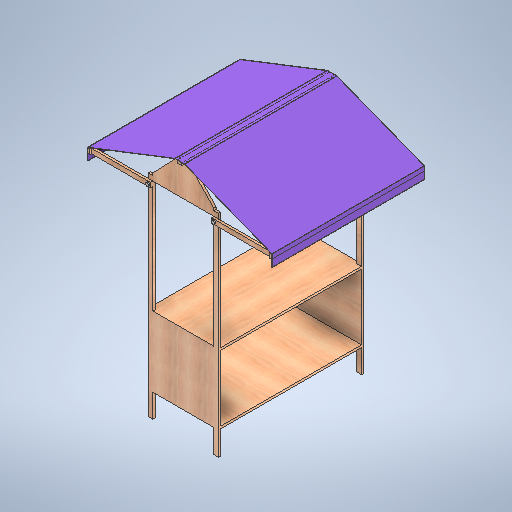
# Autodesk Inventor part: Pieza1
Saved by Autodesk Inventor 2025 (Build 290162000, 162)
## iProperties
Created: 2024-07-07
Part Number: Pieza1
Material: Genérico
Document SubType Name: Modeling
Designer: USER
Density: 1 g/cm^3
Appearance: Valor por defecto
Finish7_Appearance: Birch - Natural Medium Gloss
Finish7_Area: 449600,000 mm^2
Finish1_Appearance: Birch - Natural Polished
Finish1_Area: 7576908,613 mm^2
Finish2_Appearance: Aluminum - Polished
Finish2_Area: 5463,586 mm^2
Finish3_Appearance: Birch - Natural Polished
Finish3_Area: 400,000 mm^2
Finish4_Appearance: Birch - Natural Polished
Finish4_Area: 4880,000 mm^2
Finish5_Appearance: Birch - Natural Polished
Finish5_Area: 6080,000 mm^2
Finish6_Appearance: Violet
Finish6_Process: Prime/Paint RAL 3018
Finish6_Description: Prima/pintura RAL 3018
Finish6_ShortDescription: RAL 3018
Finish6_Thickness: 0,050 mm
Finish6_Area: 4778797,792 mm^2
Author: USER
Autodesk Inventor part; units mm, degrees
ref_plane "YZ Plane" through (0, 0, 0) normal (1, 0, 0) x (0, 1, 0)
ref_plane "XZ Plane" through (0, 0, 0) normal (0, 1, 0) x (-1, 0, 0)
ref_plane "XY Plane" through (0, 0, 0) normal (0, 0, 1) x (1, 0, 0)
sketch "Boceto1" plane through (0, 0, 0) normal (0, 1, 0) x (-1, 0, 0)
  line L0 (0, 0) -> (600, 0)
  line L1 (600, 0) -> (600, -1240)
  line L2 (600, -1240) -> (0, -1240)
  line L3 (0, -1240) -> (0, 0)
  dimension "d0" = 600
  dimension "d1" = 1240
  constraints: 8 end point, 2 parallel, 1 horizontal, 1 perpendicular
  measures "d0" distance of L1.end L2.end
  measures "d1" distance of L0.end L1.end
extrude "Extrusión1" add sketch "Boceto1" along normal blind 1800
sketch "Boceto2" plane through (-600, 0, 0) normal (0, 0, 1) x (1, 0, 0)
  line L0 (600, 0) -> (0, 0) projected
  line L1 (0, 0) -> (40, 0)
  line L2 (40, 0) -> (40, 200)
  line L3 (600, 0) -> (560, 0)
  line L4 (560, 0) -> (560, 200)
  line L5 (40, 200) -> (560, 200)
  line L6 (560, 200) -> (560, 0)
  line L7 (560, 0) -> (40, 0)
  line L8 (40, 0) -> (40, 200)
  line L9 (40, 200) -> (560, 200)
  line L10 (560, 800) -> (40, 800)
  line L11 (600, 1800) -> (0, 1800) projected
  line L12 (40, 800) -> (560, 800)
  line L13 (560, 800) -> (560, 1800)
  line L14 (560, 1800) -> (40, 1800)
  line L15 (40, 1800) -> (40, 800)
  dimension "d5" = 200
  dimension "d7" = 200
  dimension "d9" = 520
  constraints: 28 end point, 5 horizontal, 5 parallel, 4 perpendicular, 2 point on line
  measures "d5" distance of L2.end L1.end
  measures "d7" distance of L3.end L4.end
  measures "d9" distance of L14.end L13.end
extrude "Extrusión2" cut sketch "Boceto2" against normal blind 1240
sketch "Boceto3" plane through (0, 0, 0) normal (1, 0, 0) x (0, 0, -1)
  line L0 (0, 0) -> (20, 0)
  line L1 (20, 0) -> (20, 200)
  line L2 (20, 200) -> (0, 200)
  line L3 (0, 200) -> (0, 0)
  line L4 (0, 0) -> (1240, 0) projected
  line L5 (1240, 0) -> (1220, 0)
  line L6 (1220, 0) -> (1220, 200)
  line L7 (1220, 200) -> (1240, 200)
  line L8 (1240, 200) -> (1240, 0)
  line L9 (20, 200) -> (1220, 200)
  line L10 (1220, 200) -> (1220, 0)
  line L11 (1220, 0) -> (20, 0)
  line L12 (20, 0) -> (20, 200)
  line L13 (0, 800) -> (1240, 800) projected
  line L14 (20, 200) -> (1220, 200)
  line L15 (1220, 200) -> (1220, 780)
  line L16 (1220, 800) -> (20, 800)
  line L17 (20, 800) -> (20, 780)
  line L18 (20, 800) -> (1220, 800)
  line L19 (1220, 800) -> (1220, 780)
  line L20 (1220, 780) -> (20, 780)
  line L21 (20, 780) -> (20, 800)
  line L22 (20, 200) -> (1220, 200)
  line L23 (1220, 200) -> (1220, 220)
  line L24 (1220, 220) -> (20, 220)
  line L25 (20, 220) -> (20, 200)
  line L26 (0, 1800) -> (1240, 1800) projected
  line L27 (20, 800) -> (1220, 800)
  line L28 (1220, 800) -> (1220, 1800)
  line L29 (1220, 1800) -> (20, 1800)
  line L30 (20, 1800) -> (20, 800)
  line L31 (20, 780) -> (20, 220)
  line L32 (20, 220) -> (20, 200)
  line L33 (1220, 780) -> (1220, 800)
  dimension "d12" = 20
  dimension "d13" = 200
  dimension "d14" = 20
  dimension "d15" = 200
  dimension "d16" = 1200
  dimension "d17" = 20
  dimension "d18" = 1200
  dimension "d19" = 20
  dimension "d20" = 1200
  constraints: 62 end point, 19 parallel, 8 perpendicular, 7 horizontal, 2 point on line
  measures "d12" distance of L2.end L1.end
  measures "d13" distance of L1.end L0.end
  measures "d14" distance of L6.end L7.end
  measures "d15" distance of L5.end L6.end
  measures "d16" distance of L16.end L16.start
  measures "d17" distance of L18.end L15.end
  measures "d18" distance of L24.end L23.end
  measures "d19" distance of L23.end L22.end
  measures "d20" distance of L29.end L28.end
extrude "Extrusión3" cut sketch "Boceto3" against normal blind 600 contours L1 L9 L6 L4 | L30 L26 L28 L13
sketch "Boceto4" plane through (0, 0, -1240) normal (1, 0, 0) x (0, 0, -1)
  line L0 (-20, 800) -> (-20, 780)
  line L1 (-20, 780) -> (-1220, 780)
  line L2 (-1220, 780) -> (-1220, 800)
  line L3 (-20, 200) -> (-20, 220)
  line L4 (-20, 220) -> (-1220, 220)
  line L5 (-1220, 220) -> (-1220, 200)
  line L6 (-1220, 780) -> (-20, 780)
  line L7 (-20, 780) -> (-20, 220)
  line L8 (-20, 220) -> (-1220, 220)
  line L9 (-1220, 220) -> (-1220, 780)
  point P0 (-1240, 0)
  dimension "d23" = 1200
  dimension "d24" = 20
  dimension "d25" = 1200
  dimension "d26" = 20
  constraints: 20 end point, 4 parallel, 1 horizontal, 1 perpendicular
  measures "d23" distance of L0.end L1.end
  measures "d24" distance of L0.start L0.end
  measures "d25" distance of L4.end L3.end
  measures "d26" distance of L3.end L3.start
extrude "Extrusión4" cut sketch "Boceto4" against normal blind 580
sketch "Boceto5" plane through (0, 0, 0) normal (0, 0, 1) x (1, 0, 0)
  line L0 (0, 0) -> (0, 2050)
  line L1 (0, 0) -> (2050, 0) construction
  line L2 (0, 2050) -> (-560, 2050)
  line L3 (-560, 2050) -> (-560, 1760)
  line L4 (-560, 1760) -> (0, 1760)
  line L5 (0, 1760) -> (0, 2050)
  line L6 (0, 1760) -> (-40, 1760)
  line L7 (-40, 1760) -> (-40, 2050)
  line L8 (-40, 2050) -> (0, 2050)
  line L9 (0, 2050) -> (0, 1760)
  line L10 (-560, 1760) -> (-40, 1760)
  line L11 (-40, 1760) -> (-40, 1820)
  line L12 (-40, 1820) -> (-560, 1820)
  line L13 (-560, 1820) -> (-560, 1760)
  line L14 (-560, 2050) -> (-340, 2050)
  line L15 (-340, 2050) -> (-260, 2050)
  line L16 (-260, 2050) -> (-40, 1820)
  line L17 (-340, 2050) -> (-560, 1820)
  dimension "d29" = 2050
  dimension "d30" = 90
  dimension "d31" = 560
  dimension "d32" = 290
  dimension "d33" = 520
  dimension "d34" = 60
  dimension "d35" = 220
  dimension "d36" = 80
  constraints: 36 end point, 6 parallel, 4 horizontal, 4 perpendicular, 3 point on line, 1 vertical
  measures "d29" distance of L0.start L0.end
  measures "d30" angle of L1 L0
  measures "d31" distance of L4.end L3.end
  measures "d32" distance of L3.end L2.end
  measures "d33" distance of L12.end L11.end
  measures "d34" distance of L11.end L10.end
  measures "d35" distance of L2.end L14.end
  measures "d36" distance of L14.end L15.end
extrude "Extrusión5" add sketch "Boceto5" against normal blind 1240 contours L4 L3 L12 L7 | L12 L17 L2 L16
sketch "Boceto6" plane through (-40, 1760, -20) normal (1, 0, 0) x (0, 0, -1)
  line L0 (0, 0) -> (1200, 0) projected
  line L1 (-20, 290) -> (1220, 290) projected
  line L2 (0, 0) -> (1200, 0)
  line L3 (1200, 0) -> (1200, 290)
  line L4 (1200, 290) -> (0, 290)
  line L5 (0, 290) -> (0, 0)
  point P0 (-20, -1760)
  dimension "d39" = 1200
  constraints: 8 end point, 2 parallel, 1 horizontal, 1 perpendicular, 1 point on line
  measures "d39" distance of L4.end L3.end
extrude "Extrusión6" cut sketch "Boceto6" against normal blind 520
sketch "Boceto7" plane through (-600, 0, 0) normal (0, 0, 1) x (1, 0, 0)
  line L0 (40, 800) -> (40, 1760) projected
  line L1 (40, 1760) -> (-465, 1760)
  line L2 (-465, 1760) -> (-465, 1720)
  line L3 (-465, 1720) -> (40, 1720)
  line L4 (40, 1720) -> (40, 1760)
  line L5 (560, 1760) -> (560, 800) projected
  line L6 (560, 1760) -> (1065, 1760)
  line L7 (1065, 1760) -> (1065, 1720)
  line L8 (1065, 1720) -> (560, 1720)
  line L9 (560, 1720) -> (560, 1760)
  point P0 (600, 0)
  dimension "d42" = 505
  dimension "d43" = 40
  dimension "d44" = 505
  dimension "d45" = 40
  constraints: 16 end point, 4 parallel, 2 horizontal, 2 perpendicular
  measures "d42" distance of L3.end L2.end
  measures "d43" distance of L2.end L1.end
  measures "d44" distance of L7.end L8.end
  measures "d45" distance of L6.end L7.end
extrude "Extrusión7" add sketch "Boceto7" along normal blind 20 and the other way blind 1260
sketch "Boceto8" plane through (465, 1720, 20) normal (1, 0, 0) x (0, 0, -1)
  line L0 (20, 40) -> (0, 40) projected
  line L1 (1280, 0) -> (1260, 0) projected
  line L2 (20, 40) -> (1260, 40)
  line L3 (1260, 40) -> (1260, 0)
  line L4 (1260, 0) -> (20, 0)
  line L5 (20, 0) -> (20, 40)
  point P0 (20, -1720)
  constraints: 8 end point, 2 parallel, 1 horizontal, 1 perpendicular
extrude "Extrusión8" cut sketch "Boceto8" against normal blind 465
sketch "Boceto9" plane through (-1065, 1720, 20) normal (-1, 0, 0) x (0, 0, 1)
  line L0 (-20, 0) -> (-20, -920) projected
  line L1 (-1260, 40) -> (-1260, 80) projected
  line L2 (-20, 0) -> (-1260, 0)
  line L3 (-1260, 0) -> (-1260, 40)
  line L4 (-1260, 40) -> (-20, 40)
  line L5 (-20, 40) -> (-20, 0)
  point P0 (-20, -1720)
  constraints: 8 end point, 2 parallel, 1 horizontal, 1 perpendicular
extrude "Extrusión9" cut sketch "Boceto9" against normal blind 465
sketch "Boceto10" plane through (-600, 0, -1220) normal (-1, 0, 0) x (0, 0, 1)
  line L0 (0, 1760) -> (0, 1800) projected
  line L1 (0, 1720) -> (1200, 1720) projected
  line L2 (0, 1760) -> (1200, 1760)
  line L3 (1200, 1760) -> (1200, 1720)
  line L4 (1200, 1720) -> (0, 1720)
  line L5 (0, 1720) -> (0, 1760)
  point P0 (1220, 0)
  constraints: 8 end point, 2 parallel, 1 horizontal, 1 perpendicular
extrude "Extrusión10" cut sketch "Boceto10" against normal blind 600
sketch "Boceto11" plane through (-600, 0, -1260) normal (0, 0, -1) x (-1, 0, 0)
  line L0 (-560, 1760) -> (-560, 800) projected
  line L1 (-579.0242, 1739.1271) -> (-579.8656, 1739.9613)
  line L2 (-569.9328, 1749.9806) -> (-566.2222, 1736.3689)
  line L3 (-566.2222, 1736.3689) -> (-576.155, 1726.3495)
  line L4 (-576.155, 1726.3495) -> (-589.7984, 1729.9419)
  line L5 (-589.7984, 1729.9419) -> (-593.509, 1743.5536)
  line L6 (-593.509, 1743.5536) -> (-583.5762, 1753.573)
  line L7 (-583.5762, 1753.573) -> (-569.9328, 1749.9806)
  line L8 (-40, 1760) -> (-560, 1760) projected
  line L9 (0, 1760) -> (0, 1720) projected
  line L10 (-10, 1750) -> (-6.3397, 1736.3397)
  line L11 (-6.3397, 1736.3397) -> (-16.3397, 1726.3397)
  line L12 (-16.3397, 1726.3397) -> (-30, 1730)
  line L13 (-30, 1730) -> (-33.6603, 1743.6603)
  line L14 (-33.6603, 1743.6603) -> (-23.6603, 1753.6603)
  line L15 (-23.6603, 1753.6603) -> (-10, 1750)
  point P0 (-600, 0)
  point P1 (-20, 1740)
  constraints: 26 end point, 1 coincident, 26 other
extrude "Extrusión11" add sketch "Boceto11" along normal blind 10 and the other way blind 1290
sketch "Boceto12" plane through (-600, 800, -1220) normal (-1, 0, 0) x (0, 0, 1)
  line L0 (0, 1000) -> (0, 0) projected
  line L1 (1200, 960) -> (1200, 0) projected
  line L2 (0, 1000) -> (1200, 1000)
  line L3 (1200, 1000) -> (1200, 911.7503)
  line L4 (1200, 911.7503) -> (0, 911.7503)
  line L5 (0, 911.7503) -> (0, 1000)
  point P0 (1220, -800)
  constraints: 8 end point, 2 parallel, 1 horizontal, 1 perpendicular, 1 point on line
extrude "Extrusión12" cut sketch "Boceto12" against normal blind 600
sketch "Boceto13" plane through (-340, 2050, 0) normal (0, 0, 1) x (1, 0, 0)
  line L0 (-220, -230) -> (0, 0) projected
  line L1 (0, 0) -> (20, 0)
  line L2 (20, 0) -> (20, -20)
  line L3 (20, -20) -> (0, -20)
  line L4 (0, -20) -> (0, 0)
  line L5 (20, 0) -> (60, 0)
  line L6 (60, 0) -> (60, -20)
  line L7 (60, -20) -> (20, -20)
  line L8 (20, -20) -> (20, 0)
  point P0 (340, -2050)
  dimension "d62" = 20
  dimension "d63" = 20
  dimension "d64" = 40
  dimension "d65" = 20
  constraints: 16 end point, 4 parallel, 2 horizontal, 2 perpendicular
  measures "d62" distance of L2.end L3.end
  measures "d63" distance of L1.end L2.end
  measures "d64" distance of L6.end L7.end
  measures "d65" distance of L5.end L6.end
extrude "Extrusión13" add sketch "Boceto13" along normal blind 30 and the other way blind 1270 contours L5 L6 L7 L2
sketch "Boceto14" plane through (-600, 0, 20) normal (0, 0, 1) x (1, 0, 0)
  line L0 (40, 1720) -> (-465, 1720) projected
  line L1 (-465, 1720) -> (-485, 1720)
  line L2 (-485, 1720) -> (-485, 1760)
  line L3 (-485, 1760) -> (-465, 1760)
  line L4 (-465, 1760) -> (-465, 1720)
  line L5 (1065, 1760) -> (1065, 1720) projected
  line L6 (1065, 1760) -> (1085, 1760)
  line L7 (1085, 1760) -> (1085, 1720)
  line L8 (1085, 1720) -> (1065, 1720)
  line L9 (1065, 1720) -> (1065, 1760)
  point P0 (600, 0)
  dimension "d70" = 20
  dimension "d71" = 40
  dimension "d72" = 20
  constraints: 16 end point, 4 parallel, 2 horizontal, 2 perpendicular, 1 point on line
  measures "d70" distance of L2.end L3.end
  measures "d71" distance of L1.end L2.end
  measures "d72" distance of L7.end L8.end
extrude "Extrusión14" add sketch "Boceto14" along normal blind 30 and the other way blind 1290
sketch "Boceto15" plane through (485, 1720, 50) normal (1, 0, 0) x (0, 0, -1)
  line L0 (1320, 40) -> (0, 40) projected
  line L1 (1320, 0) -> (0, 0) projected
  line L2 (0, 40) -> (20, 40)
  line L3 (20, 40) -> (20, 0)
  line L4 (20, 0) -> (0, 0)
  line L5 (0, 0) -> (0, 40)
  point P0 (50, -1720)
  dimension "d77" = 20
  constraints: 8 end point, 2 parallel, 1 horizontal, 1 perpendicular, 1 point on line
  measures "d77" distance of L3.end L4.end
extrude "Extrusión15" cut sketch "Boceto15" against normal blind 1570
sketch "Boceto16" plane through (-340, 2050, 30) normal (0, 0, 1) x (1, 0, 0)
  line L0 (300, -230) -> (80, 0) projected
  line L1 (80, 0) -> (0, 0)
  line L2 (0, 3) -> (80, 3)
  line L3 (805, -290) -> (825, -290) projected
  line L4 (828, -290) -> (828, -390)
  line L5 (828, -390) -> (825, -390)
  line L6 (825, -390) -> (825, -290)
  line L7 (80, 0) -> (825, -290)
  line L8 (825, -290) -> (828, -290) construction
  line L9 (827.1213, -287.8787) -> (828, -290)
  line L10 (-745, -290) -> (-725, -290) projected
  line L11 (-748, -290) -> (-748, -390)
  line L12 (-748, -390) -> (-745, -390)
  line L13 (-745, -390) -> (-745, -290)
  line L14 (0, 0) -> (3, 0) construction
  line L15 (-2.1213, 2.1213) -> (0, 3)
  line L16 (-2.1213, 2.1213) -> (-747.1213, -287.8787)
  line L17 (-745, -290) -> (0, 0)
  line L18 (-747.1213, -287.8787) -> (-748, -290)
  line L19 (80, 0) -> (83, 0) construction
  line L20 (825, -290) -> (828, -290) construction
  line L21 (827.1213, -287.8787) -> (82.1213, 2.1213)
  line L22 (80, 3) -> (82.1213, 2.1213)
  point P0 (340, -2050)
  dimension "d80" = 80
  dimension "d81" = 3
  dimension "d82" = 3
  dimension "d83" = 100
  dimension "d84" = 3
  dimension "d87" = 3
  dimension "d88" = 100
  dimension "d89" = 3
  dimension "d90" = 3
  dimension "d92" = 3
  dimension "d94" = 3
  constraints: 40 end point, 5 horizontal, 4 parallel
  measures "d80" distance of L2.start L2.end
  measures "d81" distance of L1.end L2.start
  measures "d82" distance of L4.end L5.end
  measures "d83" distance of L4.start L4.end
  measures "d84" distance of L3.end L9.start
  measures "d87" distance of L12.end L11.end
  measures "d88" distance of L11.end L11.start
  measures "d89" distance of L10.start L16.end
  measures "d90" distance of L1.end L15.start
  measures "d92" distance of L0.end L21.end
  measures "d94" distance of L3.end L9.start
extrude "Extrusión16" add sketch "Boceto16" against normal blind 1300
sketch "Boceto17" plane through (-340, 2050, -1270) normal (0, 0, -1) x (-1, 0, 0)
  line L0 (-805, -330) -> (-805, -290) projected
  line L1 (-805, -290) -> (-825, -290)
  line L2 (-825, -290) -> (-825, -330)
  line L3 (-825, -330) -> (-805, -330)
  line L4 (-805, -330) -> (-805, -290)
  line L5 (-60, -20) -> (-20, -20) projected
  line L6 (-60, 0) -> (-20, 0)
  line L7 (-20, 0) -> (-20, -20)
  line L8 (-20, -20) -> (-60, -20)
  line L9 (-60, -20) -> (-60, 0)
  line L10 (725, -290) -> (725, -330) projected
  line L11 (745, -330) -> (745, -390) projected
  line L12 (725, -290) -> (745, -290)
  line L13 (745, -290) -> (745, -330)
  line L14 (745, -330) -> (725, -330)
  line L15 (725, -330) -> (725, -290)
  point P0 (-340, -2050)
  constraints: 24 end point, 6 parallel, 3 horizontal, 3 perpendicular
extrude "Extrusión17" add sketch "Boceto17" along normal blind 2
sketch "Boceto18" plane through (-340, 2050, 30) normal (0, 0, 1) x (1, 0, 0)
  line L0 (20, -20) -> (60, -20) projected
  line L1 (60, -20) -> (60, 0) projected
  line L2 (20, -20) -> (60, -20)
  line L3 (60, -20) -> (60, 0)
  line L4 (60, 0) -> (20, 0)
  line L5 (20, 0) -> (20, -20)
  line L6 (-745, -290) -> (-745, -330) projected
  line L7 (-725, -290) -> (-725, -330) projected
  line L8 (-745, -290) -> (-725, -290)
  line L9 (-725, -290) -> (-725, -330)
  line L10 (-725, -330) -> (-745, -330)
  line L11 (-745, -330) -> (-745, -290)
  line L12 (805, -290) -> (805, -330) projected
  line L13 (825, -390) -> (825, -330) projected
  line L14 (805, -290) -> (825, -290)
  line L15 (825, -290) -> (825, -330)
  line L16 (825, -330) -> (805, -330)
  line L17 (805, -330) -> (805, -290)
  point P0 (340, -2050)
  constraints: 24 end point, 6 parallel, 3 horizontal, 3 perpendicular
extrude "Extrusión18" add sketch "Boceto18" along normal blind 2
sketch "Boceto19" plane through (-600, 800, -1220) normal (-1, 0, 0) x (0, 0, 1)
  line L0 (295, -52.0042) -> (905, -52.0042) construction
  line L1 (905, -52.0042) -> (905, -552.7126) construction
  line L2 (905, -552.7126) -> (295, -552.7126) construction
  line L3 (295, -552.7126) -> (295, -52.0042) construction
  line L4 (-20, 0) -> (-20, 920) projected
  line L5 (-20, -800) -> (-20, 920) projected
  point P0 (905, -302.3584)
  constraints: 1 midpoint, 2 other
